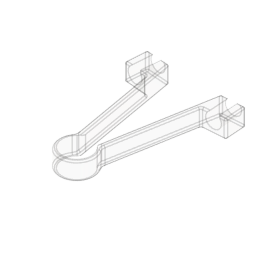
Multimeter Test Lead Tweezers (Autodesk Fusion 360 design; units mm, degrees)
Autodesk Fusion 360 part; units mm, degrees
note: some values were not read from the file. Chosen so that the rebuilt part matches the saved one: which face or edge a step refers to; which pieces of a blend or face edit are solid. Set by a fixed rule: which sketch regions a step uses.
sketch "Base Profile" plane through (0, 0, 0) normal (0, 0, 1) x (1, 0, 0) in component "Multimeter Test Lead Tweezers 8.2mm"
  circle A0 centre (0, 0) radius 8
  line L0 (0, 0) -> (0, 1.9665) construction
  line L1 (-4, 6.9282) -> (-14.3102, 65.4)
  line L2 (-14.3102, 65.4) -> (-27.2785, 66.3068)
  line L3 (-6.9857, 6.5848) -> (-15.2469, 53.4362)
  line L4 (-15.2469, 53.4362) -> (-28.1156, 54.3361)
  line L5 (-28.1156, 54.3361) -> (-27.2785, 66.3068)
  circle A1 centre (0, 0) radius 9.6
  line L6 (4, 6.9282) -> (14.3102, 65.4)
  line L7 (0, 0) -> (0, -9.6) construction
  dimension "d1" = 16
  dimension "d2" = 10
  dimension "d4" = 3
  dimension "d5" = 12
  dimension "d8" = 1.6
  dimension "d10" = 13
  dimension "d11" = 8
  dimension "d12" = 104
  dimension "d31" = 75
  constraint coincident A0.centre L0.start
  constraint vertical L0
  constraint coincident A0 L1.start
  constraint parallel L1 L3
  constraint parallel L2 L4
  constraint perpendicular L2 L5
  constraint coincident A1 L3.start
  constraint symmetric L0 L1.start L6.start
  constraint symmetric L0 L1.end L6.end
  constraint parallel L0 L7
  constraint coincident A1 L7.end
  measures "d1" diameter of A0
  measures "d2" angle of L0 L1
  measures "d4" distance of L1 L3
  measures "d5" distance of L2 L4
  measures "d8" distance of A0 A1
  measures "d10" distance of L1.end L2.end
  measures "d11" distance of L1.start L6.start
  measures "d12" angle of L3 L4
  measures "d31" vertical distance of L1.end L7.end
extrude "Extrude2" add sketch "Base Profile" along normal blind 10 contours L1 L2 L3 L4 L5 A1 makes body 1 in component "Multimeter Test Lead Tweezers 8.2mm"
sketch "Hole for Leads" plane through (3.6442, 52.1152, 0) normal (-0.069756, -0.997564, 0) x (0.997564, -0.069756, 0) in component "Multimeter Test Lead Tweezers 8.2mm"
  line L0 (-31.8374, 0) -> (-18.9373, 0)
  line L1 (-18.9373, 0) -> (-18.9373, 10)
  line L2 (-18.9373, 10) -> (-31.8374, 10)
  line L3 (-31.8374, 10) -> (-31.8374, 0)
  circle A0 centre (-25.3873, 6.7) radius 4.1
  line L4 (-25.3873, 0) -> (-25.3873, 6.7) construction
  dimension "d18" = 3.3
  dimension "d19" = 8.2
  constraint midpoint L0 L4.start
  constraint perpendicular L0 L4
  constraint coincident A0.centre L4
  constraint coincident A0.centre L4.end
  measures "d18" distance of L2 A0.centre
  measures "d19" diameter of A0
extrude "Extrude3" cut sketch "Hole for Leads" against normal up to surface (12 mm away) contours L2 A0 | L2 A0 bodies 1 in component "Multimeter Test Lead Tweezers 8.2mm"
fillet "Fillet1" radius 1 4 edges at (-15.2469, 53.4362, 5) (-28.1156, 54.3361, 5) (-14.3102, 65.4, 5) (-27.2785, 66.3068, 5) on bodies 1 in component "Multimeter Test Lead Tweezers 8.2mm"
mirror "Mirror1" about plane through (0, 0, 0) normal (1, 0, 0) of bodies 1 makes body 2 in component "Multimeter Test Lead Tweezers 8.2mm"
extrude "Extrude1" add sketch "Base Profile" along normal blind 10 contours A0 L1 A1 L6 picked at (-6.9136, 5.8313) bodies 1 2 in component "Multimeter Test Lead Tweezers 8.2mm"
fillet "Fillet3" radius 4 4 edges at (-6.9857, 6.5848, 5) (6.9857, 6.5848, 5) (4, 6.9282, 5) (-4, 6.9282, 5) on bodies 1 in component "Multimeter Test Lead Tweezers 8.2mm"
chamfer "Chamfer1" distance 0.8 angle 45 46 edges at (16.7533, 65.5708, 10) (9.2968, 36.9678, 10) (14.4902, 65.2001, 10) (-16.7533, 65.5708, 10) (-9.2968, 36.9678, 10) (-14.4902, 65.2001, 10) (11.2046, 30.511, 10) (15.4269, 53.2363, 10) (17.6402, 53.6036, 10) (-17.6402, 53.6036, 10) (-15.4269, 53.2363, 10) (-11.2046, 30.511, 10) (-7.3266, 6.8194, 10) (0, -9.6, 10) (7.3266, 6.8194, 10) (27.697, 60.3214, 10) (27.0067, 65.9942, 10) (24.7761, 66.1319, 10) (25.6132, 54.1611, 10) (27.803, 54.6078, 10) (9.2968, 36.9678, 0) (21.5721, 53.8785, 0) (27.803, 54.6078, 0) (27.697, 60.3214, 0) (27.0067, 65.9942, 0) (20.6852, 65.8458, 0) (14.4902, 65.2001, 0) (15.4269, 53.2363, 0) (-9.2968, 36.9678, 0) (-14.4902, 65.2001, 0) (-20.6852, 65.8458, 0) (-27.0067, 65.9942, 0) (-27.697, 60.3214, 0) (-27.803, 54.6078, 0) (-21.5721, 53.8785, 0) (-15.4269, 53.2363, 0) (-11.2046, 30.511, 0) (-7.3266, 6.8194, 0) (0, -9.6, 0) (7.3266, 6.8194, 0) (11.2046, 30.511, 0) (-25.6132, 54.1611, 10) (-27.803, 54.6078, 10) (-27.697, 60.3214, 10) (-27.0067, 65.9942, 10) (-24.7761, 66.1319, 10) on bodies 1 2 in component "Multimeter Test Lead Tweezers 8.2mm"
sketch "Base Profile (2)" plane through (0, 0, 0) normal (0, 0, 1) x (1, 0, 0) in component "Multimeter Test Lead Tweezers 10mm"
  circle A0 centre (0, 0) radius 8
  line L0 (0, 0) -> (0, 1.9665) construction
  line L1 (-4, 6.9282) -> (-14.3102, 65.4)
  line L2 (-14.3102, 65.4) -> (-27.2785, 66.3068)
  line L3 (-6.9857, 6.5848) -> (-15.2469, 53.4362)
  line L4 (-15.2469, 53.4362) -> (-28.1156, 54.3361)
  line L5 (-28.1156, 54.3361) -> (-27.2785, 66.3068)
  circle A1 centre (0, 0) radius 9.6
  line L6 (4, 6.9282) -> (14.3102, 65.4)
  line L7 (0, 0) -> (0, -9.6) construction
  dimension "d1_1" = 16
  dimension "d2_1" = 10
  dimension "d4_1" = 3
  dimension "d5_1" = 12
  dimension "d8_1" = 1.6
  dimension "d10_1" = 13
  dimension "d11_1" = 8
  dimension "d12_1" = 104
  dimension "d31_1" = 75
  constraint coincident A0.centre L0.start
  constraint vertical L0
  constraint coincident A0 L1.start
  constraint parallel L1 L3
  constraint parallel L2 L4
  constraint perpendicular L2 L5
  constraint coincident A1 L3.start
  constraint symmetric L0 L1.start L6.start
  constraint symmetric L0 L1.end L6.end
  constraint parallel L0 L7
  constraint coincident A1 L7.end
  measures "d1_1" diameter of A0
  measures "d2_1" angle of L0 L1
  measures "d4_1" distance of L1 L3
  measures "d5_1" distance of L2 L4
  measures "d8_1" distance of A0 A1
  measures "d10_1" distance of L1.end L2.end
  measures "d11_1" distance of L1.start L6.start
  measures "d12_1" angle of L3 L4
  measures "d31_1" vertical distance of L1.end L7.end
extrude "Extrude2'" add sketch "Base Profile (2)" along normal blind 10 separate body contours L1 L2 L3 L4 L5 A1 makes body 3 in component "Multimeter Test Lead Tweezers 10mm"
sketch "Hole for Leads (2)" plane through (3.6442, 52.1152, 0) normal (-0.069756, -0.997564, 0) x (0.997564, -0.069756, 0) in component "Multimeter Test Lead Tweezers 10mm"
  line L0 (-31.8374, 0) -> (-18.9373, 0)
  line L1 (-18.9373, 0) -> (-18.9373, 10)
  line L2 (-18.9373, 10) -> (-31.8374, 10)
  line L3 (-31.8374, 10) -> (-31.8374, 0)
  circle A0 centre (-25.3873, 7) radius 5
  line L4 (-25.3873, 0) -> (-25.3873, 7) construction
  dimension "d18_1" = 3
  dimension "d19_1" = 10
  constraint midpoint L0 L4.start
  constraint perpendicular L0 L4
  constraint coincident A0.centre L4
  constraint coincident A0.centre L4.end
  measures "d18_1" distance of L2 A0.centre
  measures "d19_1" diameter of A0
extrude "Extrude3'" cut sketch "Hole for Leads (2)" against normal up to surface (12 mm away) contours L2 A0 | L2 A0 bodies 3 in component "Multimeter Test Lead Tweezers 10mm"
fillet "Fillet1'" radius 1 4 edges at (-15.2469, 53.4362, 5) (-28.1156, 54.3361, 5) (-14.3102, 65.4, 5) (-27.2785, 66.3068, 5) on bodies 3 in component "Multimeter Test Lead Tweezers 10mm"
mirror "Mirror1'" about plane through (0, 0, 0) normal (1, 0, 0) of bodies 3 makes body 4 in component "Multimeter Test Lead Tweezers 10mm"
extrude "Extrude1'" add sketch "Base Profile (2)" along normal blind 10 contours A0 L1 A1 L6 picked at (-6.9136, 5.8313) bodies 3 4 in component "Multimeter Test Lead Tweezers 10mm"
fillet "Fillet3'" radius 4 4 edges at (-6.9857, 6.5848, 5) (6.9857, 6.5848, 5) (4, 6.9282, 5) (-4, 6.9282, 5) on bodies 3 in component "Multimeter Test Lead Tweezers 10mm"
chamfer "Chamfer1'" distance 0.8 angle 45 46 edges at (15.9717, 65.5162, 10) (9.2968, 36.9678, 10) (14.4902, 65.2001, 10) (-15.9717, 65.5162, 10) (-9.2968, 36.9678, 10) (-14.4902, 65.2001, 10) (11.2046, 30.511, 10) (15.4269, 53.2363, 10) (16.8586, 53.5489, 10) (-16.8586, 53.5489, 10) (-15.4269, 53.2363, 10) (-11.2046, 30.511, 10) (-7.3266, 6.8194, 10) (0, -9.6, 10) (7.3266, 6.8194, 10) (27.697, 60.3214, 10) (27.0067, 65.9942, 10) (25.5577, 66.1865, 10) (26.3947, 54.2157, 10) (27.803, 54.6078, 10) (9.2968, 36.9678, 0) (21.5721, 53.8785, 0) (27.803, 54.6078, 0) (27.697, 60.3214, 0) (27.0067, 65.9942, 0) (20.6852, 65.8458, 0) (14.4902, 65.2001, 0) (15.4269, 53.2363, 0) (-9.2968, 36.9678, 0) (-14.4902, 65.2001, 0) (-20.6852, 65.8458, 0) (-27.0067, 65.9942, 0) (-27.697, 60.3214, 0) (-27.803, 54.6078, 0) (-21.5721, 53.8785, 0) (-15.4269, 53.2363, 0) (-11.2046, 30.511, 0) (-7.3266, 6.8194, 0) (0, -9.6, 0) (7.3266, 6.8194, 0) (11.2046, 30.511, 0) (-26.3947, 54.2157, 10) (-27.803, 54.6078, 10) (-27.697, 60.3214, 10) (-27.0067, 65.9942, 10) (-25.5577, 66.1865, 10) on bodies 3 4 in component "Multimeter Test Lead Tweezers 10mm"
sketch "Base Profile (3)" plane through (0, 0, 0) normal (0, 0, 1) x (1, 0, 0) in component "Multimeter Test Lead Tweezers 11mm"
  circle A0 centre (0, 0) radius 8
  line L0 (0, 0) -> (0, 1.9665) construction
  line L1 (-4, 6.9282) -> (-14.3102, 65.4)
  line L2 (-14.3102, 65.4) -> (-28.2761, 66.3766)
  line L3 (-6.9857, 6.5848) -> (-15.2469, 53.4362)
  line L4 (-15.2469, 53.4362) -> (-29.1131, 54.4058)
  line L5 (-29.1131, 54.4058) -> (-28.2761, 66.3766)
  circle A1 centre (0, 0) radius 9.6
  line L6 (4, 6.9282) -> (14.3102, 65.4)
  line L7 (0, 0) -> (0, -9.6) construction
  dimension "d1_2" = 16
  dimension "d2_2" = 10
  dimension "d4_2" = 3
  dimension "d5_2" = 12
  dimension "d8_2" = 1.6
  dimension "d10_2" = 14
  dimension "d11_2" = 8
  dimension "d12_2" = 104
  dimension "d31_2" = 75
  constraint coincident A0.centre L0.start
  constraint vertical L0
  constraint coincident A0 L1.start
  constraint parallel L1 L3
  constraint parallel L2 L4
  constraint perpendicular L2 L5
  constraint coincident A1 L3.start
  constraint symmetric L0 L1.start L6.start
  constraint symmetric L0 L1.end L6.end
  constraint parallel L0 L7
  constraint coincident A1 L7.end
  measures "d1_2" diameter of A0
  measures "d2_2" angle of L0 L1
  measures "d4_2" distance of L1 L3
  measures "d5_2" distance of L2 L4
  measures "d8_2" distance of A0 A1
  measures "d10_2" distance of L1.end L2.end
  measures "d11_2" distance of L1.start L6.start
  measures "d12_2" angle of L3 L4
  measures "d31_2" vertical distance of L1.end L7.end
extrude "Extrude2''" add sketch "Base Profile (3)" along normal blind 11 separate body contours L1 L2 L3 L4 L5 A1 makes body 5 in component "Multimeter Test Lead Tweezers 11mm"
sketch "Hole for Leads (3)" plane through (3.6442, 52.1152, 0) normal (-0.069756, -0.997564, 0) x (0.997564, -0.069756, 0) in component "Multimeter Test Lead Tweezers 11mm"
  line L0 (-32.8374, 0) -> (-18.9373, 0)
  line L1 (-18.9373, 0) -> (-18.9373, 11)
  line L2 (-18.9373, 11) -> (-32.8374, 11)
  line L3 (-32.8374, 11) -> (-32.8374, 0)
  circle A0 centre (-25.8873, 8) radius 5.5
  line L4 (-25.8873, 0) -> (-25.8873, 8) construction
  dimension "d18_2" = 3
  dimension "d19_2" = 11
  constraint midpoint L0 L4.start
  constraint perpendicular L0 L4
  constraint coincident A0.centre L4
  constraint coincident A0.centre L4.end
  measures "d18_2" distance of L2 A0.centre
  measures "d19_2" diameter of A0
extrude "Extrude3''" cut sketch "Hole for Leads (3)" against normal up to surface (12 mm away) contours L2 A0 | L2 A0 bodies 5 in component "Multimeter Test Lead Tweezers 11mm"
fillet "Fillet1''" radius 1 4 edges at (-15.2469, 53.4362, 5.5) (-29.1131, 54.4058, 5.5) (-14.3102, 65.4, 5.5) (-28.2761, 66.3766, 5.5) on bodies 5 in component "Multimeter Test Lead Tweezers 11mm"
mirror "Mirror1''" about plane through (0, 0, 0) normal (1, 0, 0) of bodies 5 makes body 6 in component "Multimeter Test Lead Tweezers 11mm"
extrude "Extrude1''" add sketch "Base Profile (3)" along normal blind 11 contours A0 L1 A1 L6 picked at (-6.9136, 5.8313) bodies 5 6 in component "Multimeter Test Lead Tweezers 11mm"
fillet "Fillet3''" radius 4 4 edges at (-6.9857, 6.5848, 5.5) (6.9857, 6.5848, 5.5) (4, 6.9282, 5.5) (-4, 6.9282, 5.5) on bodies 5 in component "Multimeter Test Lead Tweezers 11mm"
chamfer "Chamfer1''" distance 0.8 angle 45 46 edges at (15.917, 65.5124, 11) (9.2968, 36.9678, 11) (14.4902, 65.2001, 11) (-15.917, 65.5124, 11) (-9.2968, 36.9678, 11) (-14.4902, 65.2001, 11) (11.2046, 30.511, 11) (15.4269, 53.2363, 11) (16.8039, 53.5451, 11) (-16.8039, 53.5451, 11) (-15.4269, 53.2363, 11) (-11.2046, 30.511, 11) (-7.3266, 6.8194, 11) (0, -9.6, 11) (7.3266, 6.8194, 11) (28.6946, 60.3912, 11) (28.0043, 66.064, 11) (26.61, 66.2601, 11) (27.4471, 54.2893, 11) (28.8005, 54.6776, 11) (9.2968, 36.9678, 0) (22.0709, 53.9134, 0) (28.8005, 54.6776, 0) (28.6946, 60.3912, 0) (28.0043, 66.064, 0) (21.184, 65.8807, 0) (14.4902, 65.2001, 0) (15.4269, 53.2363, 0) (-9.2968, 36.9678, 0) (-14.4902, 65.2001, 0) (-21.184, 65.8807, 0) (-28.0043, 66.064, 0) (-28.6946, 60.3912, 0) (-28.8005, 54.6776, 0) (-22.0709, 53.9134, 0) (-15.4269, 53.2363, 0) (-11.2046, 30.511, 0) (-7.3266, 6.8194, 0) (0, -9.6, 0) (7.3266, 6.8194, 0) (11.2046, 30.511, 0) (-27.4471, 54.2893, 11) (-28.8005, 54.6776, 11) (-28.6946, 60.3912, 11) (-28.0043, 66.064, 11) (-26.61, 66.2601, 11) on bodies 5 6 in component "Multimeter Test Lead Tweezers 11mm"
sketch "Base Profile (4)" plane through (0, 0, 0) normal (0, 0, 1) x (1, 0, 0) in component "Multimeter Test Lead Tweezers 12mm"
  circle A0 centre (0, 0) radius 8
  line L0 (0, 0) -> (0, 1.9665) construction
  line L1 (-4, 6.9282) -> (-14.3102, 65.4)
  line L2 (-14.3102, 65.4) -> (-29.2736, 66.4463)
  line L3 (-6.9857, 6.5848) -> (-15.2469, 53.4362)
  line L4 (-15.2469, 53.4362) -> (-30.1107, 54.4756)
  line L5 (-30.1107, 54.4756) -> (-29.2736, 66.4463)
  circle A1 centre (0, 0) radius 9.6
  line L6 (4, 6.9282) -> (14.3102, 65.4)
  line L7 (0, 0) -> (0, -9.6) construction
  dimension "d1_3" = 16
  dimension "d2_3" = 10
  dimension "d4_3" = 3
  dimension "d5_3" = 12
  dimension "d8_3" = 1.6
  dimension "d10_3" = 15
  dimension "d11_3" = 8
  dimension "d12_3" = 104
  dimension "d31_3" = 75
  constraint coincident A0.centre L0.start
  constraint vertical L0
  constraint coincident A0 L1.start
  constraint parallel L1 L3
  constraint parallel L2 L4
  constraint perpendicular L2 L5
  constraint coincident A1 L3.start
  constraint symmetric L0 L1.start L6.start
  constraint symmetric L0 L1.end L6.end
  constraint parallel L0 L7
  constraint coincident A1 L7.end
  measures "d1_3" diameter of A0
  measures "d2_3" angle of L0 L1
  measures "d4_3" distance of L1 L3
  measures "d5_3" distance of L2 L4
  measures "d8_3" distance of A0 A1
  measures "d10_3" distance of L1.end L2.end
  measures "d11_3" distance of L1.start L6.start
  measures "d12_3" angle of L3 L4
  measures "d31_3" vertical distance of L1.end L7.end
extrude "Extrude2'''" add sketch "Base Profile (4)" along normal blind 12 separate body contours L1 L2 L3 L4 L5 A1 makes body 7 in component "Multimeter Test Lead Tweezers 12mm"
sketch "Hole for Leads (4)" plane through (3.6442, 52.1152, 0) normal (-0.069756, -0.997564, 0) x (0.997564, -0.069756, 0) in component "Multimeter Test Lead Tweezers 12mm"
  line L0 (-33.8374, 0) -> (-18.9373, 0)
  line L1 (-18.9373, 0) -> (-18.9373, 12)
  line L2 (-18.9373, 12) -> (-33.8374, 12)
  line L3 (-33.8374, 12) -> (-33.8374, 0)
  circle A0 centre (-26.3873, 9) radius 6
  line L4 (-26.3873, 0) -> (-26.3873, 9) construction
  dimension "d18_3" = 3
  dimension "d19_3" = 12
  constraint midpoint L0 L4.start
  constraint perpendicular L0 L4
  constraint coincident A0.centre L4
  constraint coincident A0.centre L4.end
  measures "d18_3" distance of L2 A0.centre
  measures "d19_3" diameter of A0
extrude "Extrude3'''" cut sketch "Hole for Leads (4)" against normal up to surface (12 mm away) contours L2 A0 | L2 A0 bodies 7 in component "Multimeter Test Lead Tweezers 12mm"
fillet "Fillet1'''" radius 1 4 edges at (-15.2469, 53.4362, 6) (-30.1107, 54.4756, 6) (-14.3102, 65.4, 6) (-29.2736, 66.4463, 6) on bodies 7 in component "Multimeter Test Lead Tweezers 12mm"
mirror "Mirror1'''" about plane through (0, 0, 0) normal (1, 0, 0) of bodies 7 makes body 8 in component "Multimeter Test Lead Tweezers 12mm"
extrude "Extrude1'''" add sketch "Base Profile (4)" along normal blind 12 contours A0 L1 A1 L6 picked at (-6.9136, 5.8313) bodies 7 8 in component "Multimeter Test Lead Tweezers 12mm"
fillet "Fillet3'''" radius 4 4 edges at (-6.9857, 6.5848, 6) (6.9857, 6.5848, 6) (4, 6.9282, 6) (-4, 6.9282, 6) on bodies 7 in component "Multimeter Test Lead Tweezers 12mm"
chamfer "Chamfer1'''" distance 0.8 angle 45 46 edges at (15.8739, 65.5093, 12) (9.2968, 36.9678, 12) (14.4902, 65.2001, 12) (-15.8739, 65.5093, 12) (-9.2968, 36.9678, 12) (-14.4902, 65.2001, 12) (11.2046, 30.511, 12) (15.4269, 53.2363, 12) (16.7608, 53.5421, 12) (-16.7608, 53.5421, 12) (-15.4269, 53.2363, 12) (-11.2046, 30.511, 12) (-7.3266, 6.8194, 12) (0, -9.6, 12) (7.3266, 6.8194, 12) (29.6922, 60.461, 12) (29.0019, 66.1337, 12) (27.6506, 66.3329, 12) (28.4877, 54.3621, 12) (29.7981, 54.7473, 12) (9.2968, 36.9678, 0) (22.5697, 53.9483, 0) (29.7981, 54.7473, 0) (29.6922, 60.461, 0) (29.0019, 66.1337, 0) (21.6828, 65.9155, 0) (14.4902, 65.2001, 0) (15.4269, 53.2363, 0) (-9.2968, 36.9678, 0) (-14.4902, 65.2001, 0) (-21.6828, 65.9155, 0) (-29.0019, 66.1337, 0) (-29.6922, 60.461, 0) (-29.7981, 54.7473, 0) (-22.5697, 53.9483, 0) (-15.4269, 53.2363, 0) (-11.2046, 30.511, 0) (-7.3266, 6.8194, 0) (0, -9.6, 0) (7.3266, 6.8194, 0) (11.2046, 30.511, 0) (-28.4877, 54.3621, 12) (-29.7981, 54.7473, 12) (-29.6922, 60.461, 12) (-29.0019, 66.1337, 12) (-27.6506, 66.3329, 12) on bodies 7 8 in component "Multimeter Test Lead Tweezers 12mm"
sketch "Base Profile (5)" plane through (0, 0, 0) normal (0, 0, 1) x (1, 0, 0) in component "Multimeter Test Lead Tweezers 13mm"
  circle A0 centre (0, 0) radius 8
  line L0 (0, 0) -> (0, 1.9665) construction
  line L1 (-4, 6.9282) -> (-14.3102, 65.4)
  line L2 (-14.3102, 65.4) -> (-30.2712, 66.5161)
  line L3 (-6.9857, 6.5848) -> (-15.2469, 53.4362)
  line L4 (-15.2469, 53.4362) -> (-31.1083, 54.5453)
  line L5 (-31.1083, 54.5453) -> (-30.2712, 66.5161)
  circle A1 centre (0, 0) radius 9.6
  line L6 (4, 6.9282) -> (14.3102, 65.4)
  line L7 (0, 0) -> (0, -9.6) construction
  dimension "d1_4" = 16
  dimension "d2_4" = 10
  dimension "d4_4" = 3
  dimension "d5_4" = 12
  dimension "d8_4" = 1.6
  dimension "d10_4" = 16
  dimension "d11_4" = 8
  dimension "d12_4" = 104
  dimension "d31_4" = 75
  constraint coincident A0.centre L0.start
  constraint vertical L0
  constraint coincident A0 L1.start
  constraint parallel L1 L3
  constraint parallel L2 L4
  constraint perpendicular L2 L5
  constraint coincident A1 L3.start
  constraint symmetric L0 L1.start L6.start
  constraint symmetric L0 L1.end L6.end
  constraint parallel L0 L7
  constraint coincident A1 L7.end
  measures "d1_4" diameter of A0
  measures "d2_4" angle of L0 L1
  measures "d4_4" distance of L1 L3
  measures "d5_4" distance of L2 L4
  measures "d8_4" distance of A0 A1
  measures "d10_4" distance of L1.end L2.end
  measures "d11_4" distance of L1.start L6.start
  measures "d12_4" angle of L3 L4
  measures "d31_4" vertical distance of L1.end L7.end
extrude "Extrude2''''" add sketch "Base Profile (5)" along normal blind 13 separate body contours L1 L2 L3 L4 L5 A1 makes body 9 in component "Multimeter Test Lead Tweezers 13mm"
sketch "Hole for Leads (5)" plane through (3.6442, 52.1152, 0) normal (-0.069756, -0.997564, 0) x (0.997564, -0.069756, 0) in component "Multimeter Test Lead Tweezers 13mm"
  line L0 (-34.8374, 0) -> (-18.9373, 0)
  line L1 (-18.9373, 0) -> (-18.9373, 13)
  line L2 (-18.9373, 13) -> (-34.8374, 13)
  line L3 (-34.8374, 13) -> (-34.8374, 0)
  circle A0 centre (-26.8873, 10) radius 6.5
  line L4 (-26.8873, 0) -> (-26.8873, 10) construction
  dimension "d18_4" = 3
  dimension "d19_4" = 13
  constraint midpoint L0 L4.start
  constraint perpendicular L0 L4
  constraint coincident A0.centre L4
  constraint coincident A0.centre L4.end
  measures "d18_4" distance of L2 A0.centre
  measures "d19_4" diameter of A0
extrude "Extrude3''''" cut sketch "Hole for Leads (5)" against normal up to surface (12 mm away) contours L2 A0 | L2 A0 bodies 9 in component "Multimeter Test Lead Tweezers 13mm"
fillet "Fillet1''''" radius 1 4 edges at (-15.2469, 53.4362, 6.5) (-31.1083, 54.5453, 6.5) (-14.3102, 65.4, 6.5) (-30.2712, 66.5161, 6.5) on bodies 9 in component "Multimeter Test Lead Tweezers 13mm"
mirror "Mirror1''''" about plane through (0, 0, 0) normal (1, 0, 0) of bodies 9 makes body 10 in component "Multimeter Test Lead Tweezers 13mm"
extrude "Extrude1''''" add sketch "Base Profile (5)" along normal blind 13 contours A0 L1 A1 L6 picked at (-6.9136, 5.8313) bodies 9 10 in component "Multimeter Test Lead Tweezers 13mm"
fillet "Fillet3''''" radius 4 4 edges at (-6.9857, 6.5848, 6.5) (6.9857, 6.5848, 6.5) (4, 6.9282, 6.5) (-4, 6.9282, 6.5) on bodies 9 in component "Multimeter Test Lead Tweezers 13mm"
chamfer "Chamfer1''''" distance 0.8 angle 45 46 edges at (15.8389, 65.5069, 13) (9.2968, 36.9678, 13) (14.4902, 65.2001, 13) (-15.8389, 65.5069, 13) (-9.2968, 36.9678, 13) (-14.4902, 65.2001, 13) (11.2046, 30.511, 13) (15.4269, 53.2363, 13) (16.7258, 53.5396, 13) (-16.7258, 53.5396, 13) (-15.4269, 53.2363, 13) (-11.2046, 30.511, 13) (-7.3266, 6.8194, 13) (0, -9.6, 13) (7.3266, 6.8194, 13) (30.6897, 60.5307, 13) (29.9994, 66.2035, 13) (28.6832, 66.4051, 13) (29.5203, 54.4343, 13) (30.7956, 54.8171, 13) (9.2968, 36.9678, 0) (23.0685, 53.9831, 0) (30.7956, 54.8171, 0) (30.6897, 60.5307, 0) (29.9994, 66.2035, 0) (22.1816, 65.9504, 0) (14.4902, 65.2001, 0) (15.4269, 53.2363, 0) (-9.2968, 36.9678, 0) (-14.4902, 65.2001, 0) (-22.1816, 65.9504, 0) (-29.9994, 66.2035, 0) (-30.6897, 60.5307, 0) (-30.7956, 54.8171, 0) (-23.0685, 53.9831, 0) (-15.4269, 53.2363, 0) (-11.2046, 30.511, 0) (-7.3266, 6.8194, 0) (0, -9.6, 0) (7.3266, 6.8194, 0) (11.2046, 30.511, 0) (-29.5203, 54.4343, 13) (-30.7956, 54.8171, 13) (-30.6897, 60.5307, 13) (-29.9994, 66.2035, 13) (-28.6832, 66.4051, 13) on bodies 9 10 in component "Multimeter Test Lead Tweezers 13mm"
sketch "Base Profile (6)" plane through (0, 0, 0) normal (0, 0, 1) x (1, 0, 0) in component "Multimeter Test Lead Tweezers 14mm"
  circle A0 centre (0, 0) radius 8
  line L0 (0, 0) -> (0, 1.9665) construction
  line L1 (-4, 6.9282) -> (-14.3102, 65.4)
  line L2 (-14.3102, 65.4) -> (-31.7675, 66.6207)
  line L3 (-6.9857, 6.5848) -> (-15.2469, 53.4362)
  line L4 (-15.2469, 53.4362) -> (-32.6046, 54.65)
  line L5 (-32.6046, 54.65) -> (-31.7675, 66.6207)
  circle A1 centre (0, 0) radius 9.6
  line L6 (4, 6.9282) -> (14.3102, 65.4)
  line L7 (0, 0) -> (0, -9.6) construction
  dimension "d1_5" = 16
  dimension "d2_5" = 10
  dimension "d4_5" = 3
  dimension "d5_5" = 12
  dimension "d8_5" = 1.6
  dimension "d10_5" = 17.5
  dimension "d11_5" = 8
  dimension "d12_5" = 104
  dimension "d31_5" = 75
  constraint coincident A0.centre L0.start
  constraint vertical L0
  constraint coincident A0 L1.start
  constraint parallel L1 L3
  constraint parallel L2 L4
  constraint perpendicular L2 L5
  constraint coincident A1 L3.start
  constraint symmetric L0 L1.start L6.start
  constraint symmetric L0 L1.end L6.end
  constraint parallel L0 L7
  constraint coincident A1 L7.end
  measures "d1_5" diameter of A0
  measures "d2_5" angle of L0 L1
  measures "d4_5" distance of L1 L3
  measures "d5_5" distance of L2 L4
  measures "d8_5" distance of A0 A1
  measures "d10_5" distance of L1.end L2.end
  measures "d11_5" distance of L1.start L6.start
  measures "d12_5" angle of L3 L4
  measures "d31_5" vertical distance of L1.end L7.end
extrude "Extrude2'''''" add sketch "Base Profile (6)" along normal blind 14 separate body contours L1 L2 L3 L4 L5 A1 makes body 11 in component "Multimeter Test Lead Tweezers 14mm"
sketch "Hole for Leads (6)" plane through (3.6442, 52.1152, 0) normal (-0.069756, -0.997564, 0) x (0.997564, -0.069756, 0) in component "Multimeter Test Lead Tweezers 14mm"
  line L0 (-36.3374, 0) -> (-18.9373, 0)
  line L1 (-18.9373, 0) -> (-18.9373, 14)
  line L2 (-18.9373, 14) -> (-36.3374, 14)
  line L3 (-36.3374, 14) -> (-36.3374, 0)
  circle A0 centre (-27.6373, 10.5) radius 7
  line L4 (-27.6373, 0) -> (-27.6373, 10.5) construction
  dimension "d18_5" = 3.5
  dimension "d19_5" = 14
  constraint midpoint L0 L4.start
  constraint perpendicular L0 L4
  constraint coincident A0.centre L4
  constraint coincident A0.centre L4.end
  measures "d18_5" distance of L2 A0.centre
  measures "d19_5" diameter of A0
extrude "Extrude3'''''" cut sketch "Hole for Leads (6)" against normal up to surface (12 mm away) contours L2 A0 | L2 A0 bodies 11 in component "Multimeter Test Lead Tweezers 14mm"
fillet "Fillet1'''''" radius 1 4 edges at (-15.2469, 53.4362, 7) (-32.6046, 54.65, 7) (-14.3102, 65.4, 7) (-31.7675, 66.6207, 7) on bodies 11 in component "Multimeter Test Lead Tweezers 14mm"
mirror "Mirror1'''''" about plane through (0, 0, 0) normal (1, 0, 0) of bodies 11 makes body 12 in component "Multimeter Test Lead Tweezers 14mm"
extrude "Extrude1'''''" add sketch "Base Profile (6)" along normal blind 14 contours A0 L1 A1 L6 picked at (-6.9136, 5.8313) bodies 11 12 in component "Multimeter Test Lead Tweezers 14mm"
fillet "Fillet3'''''" radius 4 4 edges at (-6.9857, 6.5848, 7) (6.9857, 6.5848, 7) (4, 6.9282, 7) (-4, 6.9282, 7) on bodies 11 in component "Multimeter Test Lead Tweezers 14mm"
chamfer "Chamfer1'''''" distance 0.8 angle 45 46 edges at (16.0654, 65.5227, 14) (9.2968, 36.9678, 14) (14.4902, 65.2001, 14) (-16.0654, 65.5227, 14) (-9.2968, 36.9678, 14) (-14.4902, 65.2001, 14) (11.2046, 30.511, 14) (15.4269, 53.2363, 14) (16.9523, 53.5555, 14) (-16.9523, 53.5555, 14) (-15.4269, 53.2363, 14) (-11.2046, 30.511, 14) (-7.3266, 6.8194, 14) (0, -9.6, 14) (7.3266, 6.8194, 14) (32.1861, 60.6354, 14) (31.4958, 66.3081, 14) (29.953, 66.4939, 14) (30.7901, 54.5231, 14) (32.292, 54.9217, 14) (9.2968, 36.9678, 0) (23.8167, 54.0355, 0) (32.292, 54.9217, 0) (32.1861, 60.6354, 0) (31.4958, 66.3081, 0) (22.9298, 66.0027, 0) (14.4902, 65.2001, 0) (15.4269, 53.2363, 0) (-9.2968, 36.9678, 0) (-14.4902, 65.2001, 0) (-22.9298, 66.0027, 0) (-31.4958, 66.3081, 0) (-32.1861, 60.6354, 0) (-32.292, 54.9217, 0) (-23.8167, 54.0355, 0) (-15.4269, 53.2363, 0) (-11.2046, 30.511, 0) (-7.3266, 6.8194, 0) (0, -9.6, 0) (7.3266, 6.8194, 0) (11.2046, 30.511, 0) (-30.7901, 54.5231, 14) (-32.292, 54.9217, 14) (-32.1861, 60.6354, 14) (-31.4958, 66.3081, 14) (-29.953, 66.4939, 14) on bodies 11 12 in component "Multimeter Test Lead Tweezers 14mm"
sketch "Base Profile (7)" plane through (0, 0, 0) normal (0, 0, 1) x (1, 0, 0) in component "Multimeter Test Lead Tweezers 15mm"
  circle A0 centre (0, 0) radius 8
  line L0 (0, 0) -> (0, 1.9665) construction
  line L1 (-4, 6.9282) -> (-14.3102, 65.4)
  line L2 (-14.3102, 65.4) -> (-32.7651, 66.6905)
  line L3 (-6.9857, 6.5848) -> (-15.2469, 53.4362)
  line L4 (-15.2469, 53.4362) -> (-33.6022, 54.7197)
  line L5 (-33.6022, 54.7197) -> (-32.7651, 66.6905)
  circle A1 centre (0, 0) radius 9.6
  line L6 (4, 6.9282) -> (14.3102, 65.4)
  line L7 (0, 0) -> (0, -9.6) construction
  dimension "d1_6" = 16
  dimension "d2_6" = 10
  dimension "d4_6" = 3
  dimension "d5_6" = 12
  dimension "d8_6" = 1.6
  dimension "d10_6" = 18.5
  dimension "d11_6" = 8
  dimension "d12_6" = 104
  dimension "d31_6" = 75
  constraint coincident A0.centre L0.start
  constraint vertical L0
  constraint coincident A0 L1.start
  constraint parallel L1 L3
  constraint parallel L2 L4
  constraint perpendicular L2 L5
  constraint coincident A1 L3.start
  constraint symmetric L0 L1.start L6.start
  constraint symmetric L0 L1.end L6.end
  constraint parallel L0 L7
  constraint coincident A1 L7.end
  measures "d1_6" diameter of A0
  measures "d2_6" angle of L0 L1
  measures "d4_6" distance of L1 L3
  measures "d5_6" distance of L2 L4
  measures "d8_6" distance of A0 A1
  measures "d10_6" distance of L1.end L2.end
  measures "d11_6" distance of L1.start L6.start
  measures "d12_6" angle of L3 L4
  measures "d31_6" vertical distance of L1.end L7.end
extrude "Extrude2''''''" add sketch "Base Profile (7)" along normal blind 15.5 separate body contours L1 L2 L3 L4 L5 A1 makes body 13 in component "Multimeter Test Lead Tweezers 15mm"
sketch "Hole for Leads (7)" plane through (3.6442, 52.1152, 0) normal (-0.069756, -0.997564, 0) x (0.997564, -0.069756, 0) in component "Multimeter Test Lead Tweezers 15mm"
  line L0 (-37.3374, 0) -> (-18.9373, 0)
  line L1 (-18.9373, 0) -> (-18.9373, 15.5)
  line L2 (-18.9373, 15.5) -> (-37.3374, 15.5)
  line L3 (-37.3374, 15.5) -> (-37.3374, 0)
  circle A0 centre (-28.1373, 10.5) radius 7.5
  line L4 (-28.1373, 0) -> (-28.1373, 10.5) construction
  dimension "d18_6" = 5
  dimension "d19_6" = 15
  constraint midpoint L0 L4.start
  constraint perpendicular L0 L4
  constraint coincident A0.centre L4
  constraint coincident A0.centre L4.end
  measures "d18_6" distance of L2 A0.centre
  measures "d19_6" diameter of A0
extrude "Extrude3''''''" cut sketch "Hole for Leads (7)" against normal up to surface (12 mm away) contours L2 A0 | L2 A0 bodies 13 in component "Multimeter Test Lead Tweezers 15mm"
fillet "Fillet1''''''" radius 1 4 edges at (-15.2469, 53.4362, 7.75) (-33.6022, 54.7197, 7.75) (-14.3102, 65.4, 7.75) (-32.7651, 66.6905, 7.75) on bodies 13 in component "Multimeter Test Lead Tweezers 15mm"
mirror "Mirror1''''''" about plane through (0, 0, 0) normal (1, 0, 0) of bodies 13 makes body 14 in component "Multimeter Test Lead Tweezers 15mm"
extrude "Extrude1''''''" add sketch "Base Profile (7)" along normal blind 15.5 contours A0 L1 A1 L6 picked at (-6.9136, 5.8313) bodies 13 14 in component "Multimeter Test Lead Tweezers 15mm"
fillet "Fillet3''''''" radius 4 4 edges at (-6.9857, 6.5848, 7.75) (6.9857, 6.5848, 7.75) (4, 6.9282, 7.75) (-4, 6.9282, 7.75) on bodies 13 in component "Multimeter Test Lead Tweezers 15mm"
chamfer "Chamfer1''''''" distance 0.8 angle 45 46 edges at (16.5502, 65.5566, 15.5) (9.2968, 36.9678, 15.5) (14.4902, 65.2001, 15.5) (-16.5502, 65.5566, 15.5) (-9.2968, 36.9678, 15.5) (-14.4902, 65.2001, 15.5) (11.2046, 30.511, 15.5) (15.4269, 53.2363, 15.5) (17.4371, 53.5894, 15.5) (-17.4371, 53.5894, 15.5) (-15.4269, 53.2363, 15.5) (-11.2046, 30.511, 15.5) (-7.3266, 6.8194, 15.5) (0, -9.6, 15.5) (7.3266, 6.8194, 15.5) (33.1836, 60.7051, 15.5) (32.4933, 66.3779, 15.5) (30.4658, 66.5297, 15.5) (31.3028, 54.5589, 15.5) (33.2896, 54.9915, 15.5) (9.2968, 36.9678, 0) (24.3154, 54.0703, 0) (33.2896, 54.9915, 0) (33.1836, 60.7051, 0) (32.4933, 66.3779, 0) (23.4285, 66.0376, 0) (14.4902, 65.2001, 0) (15.4269, 53.2363, 0) (-9.2968, 36.9678, 0) (-14.4902, 65.2001, 0) (-23.4285, 66.0376, 0) (-32.4933, 66.3779, 0) (-33.1836, 60.7051, 0) (-33.2896, 54.9915, 0) (-24.3154, 54.0703, 0) (-15.4269, 53.2363, 0) (-11.2046, 30.511, 0) (-7.3266, 6.8194, 0) (0, -9.6, 0) (7.3266, 6.8194, 0) (11.2046, 30.511, 0) (-31.3028, 54.5589, 15.5) (-33.2896, 54.9915, 15.5) (-33.1836, 60.7051, 15.5) (-32.4933, 66.3779, 15.5) (-30.4658, 66.5297, 15.5) on bodies 13 14 in component "Multimeter Test Lead Tweezers 15mm"
component "Multimeter Test Lead Tweezers 8.2mm" placed x (1, 0, 0) y (0, 1, 0) z (0, 0, 1) at (0, 0, 0)
component "Multimeter Test Lead Tweezers 10mm" placed x (1, 0, 0) y (0, 1, 0) z (0, 0, 1) at (0, 0, 0)
component "Multimeter Test Lead Tweezers 11mm" placed x (1, 0, 0) y (0, 1, 0) z (0, 0, 1) at (0, 0, 0)
component "Multimeter Test Lead Tweezers 12mm" placed x (1, 0, 0) y (0, 1, 0) z (0, 0, 1) at (0, 0, 0)
component "Multimeter Test Lead Tweezers 13mm" placed x (1, 0, 0) y (0, 1, 0) z (0, 0, 1) at (0, 0, 0)
component "Multimeter Test Lead Tweezers 14mm" placed x (1, 0, 0) y (0, 1, 0) z (0, 0, 1) at (0, 0, 0)
component "Multimeter Test Lead Tweezers 15mm" placed x (1, 0, 0) y (0, 1, 0) z (0, 0, 1) at (0, 0, 0)
component "Multimeter Test Lead Tweezers 8.2mm" placed x (1, 0, 0) y (0, 1, 0) z (0, 0, 1) at (0, 0, 0)
named bodies: "8.2mm Multimeter Test Lead Tweezers", "10mm Multimeter Test Lead Tweezers", "11mm Multimeter Test Lead Tweezers", "12mm Multimeter Test Lead Tweezers", "13mm Multimeter Test Lead Tweezers", "14 mm Multimeter Test Lead Tweezers", "15mm Multimeter Test Lead Tweezers"
